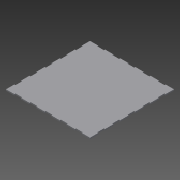
# Autodesk Inventor part: wordClock
Saved by Autodesk Inventor 2015 (Build 190159000, 159)
## iProperties
Created: 2015-02-10
Part Number: wordClock
Material: Generic
Document SubType Name: Modeling
Designer: Iain
Density: 1 g/cm^3
Appearance: Default
Author: Iain
Autodesk Inventor part; units mm, degrees
ref_plane "YZ Plane" through (0, 0, 0) normal (1, 0, 0) x (0, 1, 0)
ref_plane "XZ Plane" through (0, 0, 0) normal (0, 1, 0) x (-1, 0, 0)
ref_plane "XY Plane" through (0, 0, 0) normal (0, 0, 1) x (1, 0, 0)
sketch "Sketch1" plane through (0, 0, 0) normal (0, 0, 1) x (1, 0, 0)
  line L0 (-97, 97) -> (97, 97)
  line L1 (97, 97) -> (97, -97)
  line L2 (97, -97) -> (-97, -97)
  line L3 (-97, -97) -> (-97, 97)
  point P0 (0, 0)
  point P1 (0, 97)
  point P2 (-97, 0)
  dimension "FrontFaceWidth" = 194
  dimension "FrontFaceHeight" = 194
  constraints: 8 end point, 2 midpoint, 2 parallel, 1 horizontal, 1 horizontal alignment, 1 perpendicular, 1 vertical alignment
  measures "FrontFaceWidth" distance of L0.start L0.end
  measures "FrontFaceHeight" distance of L2.end L0.start
extrude "Extrusion1" add sketch "Sketch1" along normal mid plane 3
sketch "Sketch4" plane through (0, 0, 1.5) normal (0, 0, 1) x (1, 0, 0)
  line L0 (-100, 100) -> (-80, 100)
  line L1 (-80, 100) -> (-80, 97)
  line L2 (-80, 97) -> (-100, 97)
  line L3 (-100, 97) -> (-100, 100)
  point P0 (-97, 97)
  point P1 (0, 0)
  point P2 (-90, 97)
  dimension "d6" = 3
  dimension "FrontFaceTabWidth" = 20
  dimension "d8" = 3
  constraints: 8 end point, 2 parallel, 1 horizontal, 1 horizontal alignment, 1 midpoint, 1 perpendicular
  measures "d6" distance of point (-97, 97) L2.end
  measures "FrontFaceTabWidth" distance of L0.end L0.start
  measures "d8" distance of L1.end L0.end
extrude "Extrusion2" add sketch "Sketch4" against normal blind 3
pattern_linear "FrontTopTabs" count 6 spacing 36 along (1, 0, 0) of "Extrusion2"
sketch "Sketch5" plane through (0, 0, 1.5) normal (0, 0, 1) x (1, 0, 0)
  line L0 (-100, -100) -> (-97, -100)
  line L1 (-97, -100) -> (-97, -80)
  line L2 (-97, -80) -> (-100, -80)
  line L3 (-100, -80) -> (-100, -100)
  point P0 (-97, -97)
  point P1 (0, 0)
  point P2 (-97, -90)
  dimension "d14" = 3
  dimension "d15" = 3
  dimension "d16" = 20
  constraints: 8 end point, 2 parallel, 1 horizontal, 1 midpoint, 1 perpendicular, 1 vertical alignment
  measures "d14" distance of point (-97, -97) L0.end
  measures "d15" distance of L0.start L0.end
  measures "d16" distance of L2.end L0.start
extrude "Extrusion3" add sketch "Sketch5" against normal blind 3
pattern_linear "FontLeftTabs" count 6 spacing 36 along (0, 1, 0) of "Extrusion3"
mirror "FrontBottomTabs" about plane through (0, 0, 0) normal (0, 1, 0) of "Extrusion2", "FrontTopTabs"
mirror "FontRightTabs" about plane through (0, 0, 0) normal (1, 0, 0) of "Extrusion3", "FontLeftTabs"
equation "\"FrontFaceWidth\" = ClockWidth - 2 * FrontFaceTabDepth"
equation "\"FrontFaceHeight\" = ClockHeight - 2 * FrontFaceTabDepth"
equation "\"FrontFaceThickness\" = Ply3mm"
equation "\"d6\" = TabDepth"
equation "\"d8\" = FrontFaceTabDepth"
equation "\"d9\" = FrontFaceThickness"
equation "\"d14\" = FrontFaceTabDepth"
equation "\"d15\" = FrontFaceTabDepth"
equation "\"d16\" = FrontFaceTabWidth"
equation "\"d17\" = FrontFaceThickness"
equation "\"FrontFaceTabDepth\" = TabDepth"
equation "\"Ply3mm\" = 3"
equation "\"TabDepth\" = Ply3mm"
equation "\"ClockWidth\" = 200"
equation "\"ClockHeight\" = 200"
